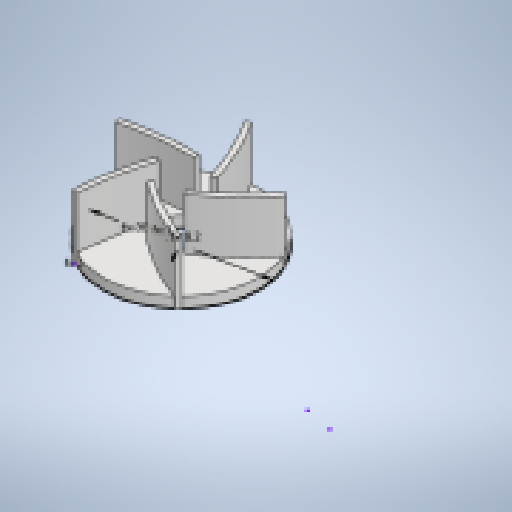
# Autodesk Inventor part: Propeller
Saved by Autodesk Inventor 2023.1 (Build 271208000, 208)
## iProperties
Created: 2024-02-14
Part Number: Propeller
Material: Generic
Document SubType Name: Modeling
Designer: USER
Density: 1 g/cm^3
Appearance: Default
Author: USER
Autodesk Inventor part; units mm, degrees
ref_plane "YZ Plane" through (0, 0, 0) normal (1, 0, 0) x (0, 1, 0)
ref_plane "XZ Plane" through (0, 0, 0) normal (0, 1, 0) x (-1, 0, 0)
ref_plane "XY Plane" through (0, 0, 0) normal (0, 0, 1) x (1, 0, 0)
sketch "Sketch1" plane through (0, 0, 0) normal (0, 1, 0) x (-1, 0, 0)
  circle A0 centre (0, 0) radius 15
  circle A1 centre (0, 0) radius 4.1
  arc A2 (4.1, 0) -> (6.6908, 13.4251) centre (-45.2629, 16.4886) ccw
  line L0 (4.1, 0) -> (5.0548, -0.2974)
  line L1 (6.6908, 13.4251) -> (7.6829, 13.2996)
  arc A3 (5.0548, -0.2974) -> (7.6829, 13.2996) centre (-40.0035, 15.4643) ccw
  dimension "d0" = 30
  dimension "d1" = 8.2
  dimension "d10" = 1
  dimension "d11" = 1
  constraints: 4 end point, 4 point on circle, 2 centre point, 2 coincident, 6 other
  measures "d10" distance of L0.start L0.end
  measures "d11" distance of L1.start L1.end
extrude "Extrusion1" add sketch "Sketch1" along normal blind 2 contours A2 L0 A3 A0 | A0 A3 L0 A2
extrude "Extrusion3" add sketch "Sketch1" along normal blind 12 contours L1 A3 A0 | A0 A3 L0 A2 picked at (6.2625, 7.2317)
pattern_circular "Circular Pattern2" count 6 over 360 about axis through (0, 0, 0) along (0, 1, 0) of "Extrusion3"
equation "\"d0\" = PropDiameter"
equation "\"d1\" = PropHoleDiameter"
equation "\"d10\" = PropBladeThickness"
equation "\"d11\" = PropBladeThickness"
equation "\"d2\" = PropPlateThickness"
equation "\"d12\" = PropPlateThickness + PropDepth"
equation "\"PropHoleDiameter\" = 8.2"
equation "\"PropDepth\" = 10"
equation "\"PropPlateThickness\" = 2"
equation "\"PropBladeThickness\" = 1"
equation "\"VoluteCaseInnerSize\" = 31"
equation "\"VoluteCaseOuterSize\" = 42"
equation "\"VoluteWallThickness\" = 2"
equation "\"VoluteStartAngle\" = 25deg"
equation "\"PropDiameter\" = 30"
body "Solid1"
